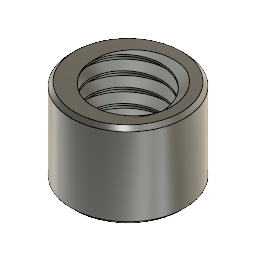
cnc halterung schutzkappe v1 (Autodesk Fusion 360 design; units mm, degrees)
Autodesk Fusion 360 part; units mm, degrees
note: some values were not read from the file. Set by a fixed rule: which face or edge a step refers to.
sketch "Skizze1" plane through (0, 0, 0) normal (0, 0, 1) x (1, 0, 0)
  circle A0 centre (0, 0) radius 3
  dimension "d1" = 6
  measures "d1" diameter of A0
extrude "Extrusion1" add sketch "Skizze1" along normal blind 5
shell "Schale1" thickness 1 outward yes removed faces 1 at (-1.1591, 0.5829, 5)
thread "Gewinde1" "ISO Metric profile 6.0 M6x1 6H" major diameter 6.147 minor diameter 5.035 pitch 1 angle 60 modelled right hand crest width 0.125 on face at (2.9963, -0.1495, 3.3333) crest through (2.5175, 0, -0.5625)
chamfer "Fase1" distance 0.25 angle 45 2 edges at (-3.7293, -1.4465, -1) (-3.7293, -1.4465, 5)
